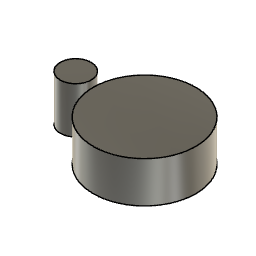
3mm 10mm v1 v1 v1 (Autodesk Fusion 360 design; units mm, degrees)
Autodesk Fusion 360 part; units mm, degrees
sketch "Sketch1" plane through (0, 0, 0) normal (0, 0, 1) x (1, 0, 0)
  circle A0 centre (2.2778, 0) radius 1.5
  circle A1 centre (9, 0) radius 5
  dimension "d1" = 3
  dimension "d2" = 10
  measures "d1" diameter of A0
  measures "d2" diameter of A1
extrude "Extrude1" add sketch "Sketch1" along normal blind 2 makes body 1 at (10.3101, -1.9935, 0) makes body 2 at (3.7759, -0.0748, 1.3333)
extrude "Extrude2" add 1 faces at (2.7283, -0.3464, 2) along direction (0, 0, 1) blind 2.5 on bodies 2 bodies 2
extrude "Extrude3" add 1 faces at (10.3101, -1.9935, 2) along direction (0, 0, 1) blind 2 on bodies 1 bodies 1
